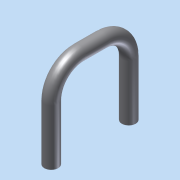
# Autodesk Inventor part: antenna_stop_3
Saved by Autodesk Inventor 2014 SP1 (Build 180222100, 222)
## iProperties
Created: 2013-09-08
Part Number: antenna_stop_3
Document SubType Name: Modeling
Designer: Robert Davis
Density: 1 g/cm^3
Material: Generic
Appearance: Default
Author: Robert Davis
Autodesk Inventor part; units mm, degrees
ref_plane "YZ Plane" through (0, 0, 0) normal (1, 0, 0) x (0, 1, 0)
ref_plane "XZ Plane" through (0, 0, 0) normal (0, 1, 0) x (-1, 0, 0)
ref_plane "XY Plane" through (0, 0, 0) normal (0, 0, 1) x (1, 0, 0)
sketch "Sketch1" plane through (0, 0, 0) normal (0, 0, 1) x (1, 0, 0)
  circle A0 centre (0, 0) radius 0.25
  dimension "d0" = 0.5
  constraints: 1 centre point
  measures "d0" diameter of A0
sketch3d "3D Sketch2"
  line L0 (0, 0, 0) -> (0, 0, 1.9964)
  arc A0 (0, 0, 1.9964) -> (0, 1.0036, 2.9964) centre (0, 1, 1.9964) ccw
  line L1 (0, 1.0036, 2.9964) -> (0, 1.7985, 2.9936)
  arc A1 (0, 1.7985, 2.9936) -> (0, 2.795, 1.9936) centre (0, 1.795, 1.9936) ccw
  line L2 (0, 2.795, 1.9936) -> (0, 2.795, -0.01)
  dimension "d8" = 3
  dimension "d9" = 2.795
  dimension "d10" = 3
  dimension "d5" = 1
  dimension "d6" = 1
  constraints: 4 horizontal
sweep "Sweep1" add profiles "Sketch1" path "3D Sketch2"
equation "\"d6\" = d5"
body "Solid1"
